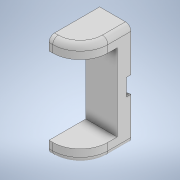
# Autodesk Inventor part: Spine
Saved by Autodesk Inventor 2022 (Build 260153000, 153)
## iProperties
Created: 2022-05-09
Part Number: Spine
Material: Generic
Document SubType Name: Modeling
Designer: dirks
Density: 1 g/cm^3
Appearance: Default
Author: dirks
Autodesk Inventor part; units mm, degrees
ref_plane "YZ Plane" through (0, 0, 0) normal (1, 0, 0) x (0, 1, 0)
ref_plane "XZ Plane" through (0, 0, 0) normal (0, 1, 0) x (-1, 0, 0)
ref_plane "XY Plane" through (0, 0, 0) normal (0, 0, 1) x (1, 0, 0)
sketch "Sketch10" plane through (0, 0, 0) normal (0, 0, 1) x (1, 0, 0)
  line L0 (0, 0) -> (17, 0)
  line L1 (17, 0) -> (17, 55)
  line L2 (17, 55) -> (0, 55)
  line L3 (0, 55) -> (0, 0)
  dimension "d24" = 17
  dimension "d25" = 55
  constraints: 8 end point, 2 parallel, 1 horizontal, 1 perpendicular
  measures "d24" distance of L2.end L1.end
  measures "d25" distance of L1.end L0.end
extrude "Extrusion9" add sketch "Sketch10" along normal blind 5
sketch "Sketch12" plane through (0, 0, 5) normal (0, 0, 1) x (1, 0, 0)
  line L0 (17, 0) -> (17, 55) projected
  line L1 (0, 55) -> (0, 0) projected
  line L2 (0, 0) -> (17, 0) projected
  line L3 (0, 0) -> (17, 0)
  line L4 (17, 0) -> (17, 6)
  line L5 (17, 6) -> (0, 6)
  line L6 (0, 6) -> (0, 0)
  dimension "d32" = 17
  dimension "d33" = 6
  constraints: 8 end point, 2 parallel, 1 horizontal, 1 perpendicular
  measures "d32" distance of L5.end L4.end
  measures "d33" distance of L4.end L3.end
extrude "Extrusion11" add sketch "Sketch12" along normal blind 20
sketch "Sketch13" plane through (0, 0, 0) normal (0, -1, 0) x (1, 0, 0)
  line L0 (0, 0) -> (17, 0) projected
  line L1 (17, 0) -> (17, 25) projected
  line L2 (0, 25) -> (17, 25) projected
  line L3 (0, 0) -> (0, 25) projected
extrude "Extrusion12" add sketch "Sketch13" along normal blind 1
sketch "Sketch14" plane through (0, 0, 5) normal (0, 0, 1) x (1, 0, 0)
  line L0 (17, 6) -> (17, 55) projected
  line L1 (17, 55) -> (0, 55) projected
  line L2 (0, 55) -> (0, 6) projected
  line L3 (17, 55) -> (0, 55) projected
  line L4 (0, 55) -> (17, 55)
  line L5 (17, 55) -> (17, 48)
  line L6 (17, 48) -> (0, 48)
  line L7 (0, 48) -> (0, 55)
  point P0 (0, 0)
  dimension "d38" = 17
  dimension "d39" = 7
  constraints: 8 end point, 2 parallel, 1 horizontal, 1 perpendicular
  measures "d38" distance of L5.end L6.end
  measures "d39" distance of L4.end L5.end
extrude "Extrusion13" add sketch "Sketch14" along normal up to surface (20 mm away)
fillet "Fillet1" radius 15 1 edges at (17, 51.5, 25)
fillet "Fillet2" radius 15 1 edges at (17, 2.5, 25)
fillet "Fillet3" radius 3 3 edges at (1, 55, 25) (17, 55, 5) (12.6066, 55, 20.6066)
fillet "Fillet4" radius 3 3 edges at (12.6066, -1, 20.6066) (1, -1, 25) (17, -1, 5)
sketch "Sketch15" plane through (0, 0, 0) normal (0, 0, -1) x (-1, 0, 0)
  arc A0 (-17, 2) -> (-14, -1) centre (-14, 2) ccw projected
  line L0 (0, -1) -> (-14, -1) projected
  line L1 (0, 55) -> (0, -1) projected
  line L2 (-14, 55) -> (0, 55) projected
  arc A1 (-14, 55) -> (-17, 52) centre (-14, 52) ccw projected
  line L3 (-17, 2) -> (-17, 52) projected
  line L4 (8.7827, 30.0642) -> (-3.3501, 32.1768) projected
  line L5 (-5.4735, 44.3389) -> (-3.3501, 32.1768) projected
  line L6 (-5.4735, 44.3389) -> (-5.8165, 45.0526) projected
  line L7 (-5.8165, 45.0526) -> (-6.5415, 45.6348) projected
  line L8 (-7.5479, 46.0014) -> (-6.5415, 45.6348) projected
  line L9 (-8.6908, 46.1) -> (-7.5479, 46.0014) projected
  line L10 (-8.6908, 46.1) -> (-9.8101, 45.9193) projected
  line L11 (-9.8101, 45.9193) -> (-10.7456, 45.4818) projected
  line L12 (-11.3668, 44.8513) -> (-10.7456, 45.4818) projected
  line L13 (-11.564, 44.3389) -> (-13.6922, 32.1494) projected
  line L14 (-11.3668, 44.8513) -> (-11.564, 44.3389) projected
  line L15 (-13.6922, 32.1494) -> (-25.8859, 30.0262) projected
  line L16 (-25.8859, 23.9358) -> (-13.6462, 21.8046) projected
  line L17 (-3.3041, 21.8692) -> (-5.4356, 9.6611) projected
  line L18 (8.7827, 23.9738) -> (-3.3041, 21.8692) projected
  line L19 (-13.6462, 21.8046) -> (-11.526, 9.6611) projected
  line L20 (-11.526, 9.6611) -> (-11.183, 8.9474) projected
  line L21 (-11.183, 8.9474) -> (-10.458, 8.3652) projected
  line L22 (-10.458, 8.3652) -> (-9.4517, 7.9986) projected
  line L23 (-9.4517, 7.9986) -> (-8.3088, 7.9) projected
  line L24 (-8.3088, 7.9) -> (-7.1895, 8.0807) projected
  line L25 (-7.1895, 8.0807) -> (-6.254, 8.5182) projected
  line L26 (-6.254, 8.5182) -> (-5.6327, 9.1487) projected
  line L27 (-5.4356, 9.6611) -> (-5.6327, 9.1487) projected
  line L28 (0, 48) -> (0, 6) projected
  line L29 (0, 31.5935) -> (-3.3501, 32.1768)
  line L30 (-3.3501, 32.1768) -> (-5.4735, 44.3389)
  line L31 (-3.3041, 21.8692) -> (0, 22.4445)
  line L32 (-3.3041, 21.8692) -> (-5.4356, 9.6611)
  line L33 (-11.526, 9.6611) -> (-13.6462, 21.8046)
  line L34 (-13.6462, 21.8046) -> (-17, 22.3886)
  line L35 (-17, 6) -> (-17, 48) projected
  line L36 (-17, 31.5735) -> (-13.6922, 32.1494)
  line L37 (-13.6922, 32.1494) -> (-11.564, 44.3389)
  arc A2 (-5.4735, 44.3389) -> (-11.564, 44.3389) centre (-8.5188, 42.5301) ccw
  arc A3 (-11.526, 9.6611) -> (-5.4356, 9.6611) centre (-8.4808, 11.4699) ccw
  line L38 (0, 31.5935) -> (0, 22.4445)
  line L39 (-17, 22.3886) -> (-17, 31.5735)
  line L40 (0, 55) -> (0, 52) projected
  line L41 (0, 31.5935) -> (0, 55)
  line L42 (0, 55) -> (-14, 55)
  line L43 (0, 22.4445) -> (0, -1)
  line L44 (-2, -1) -> (-14, -1) projected
  line L45 (-14, -1) -> (0, -1)
  line L46 (-17, 2) -> (-17, 6) projected
  line L47 (-17, 2) -> (-17, 22.3886)
  line L48 (-17, 31.5735) -> (-17, 48)
  arc A4 (-14, 55) -> (-17, 52) centre (-14, 52) ccw
  arc A5 (-17, 2) -> (-14, -1) centre (-14, 2) ccw
  line L49 (-17, 48) -> (-17, 52)
  point P0 (0, 0)
  point P1 (0, 22.4445)
  point P2 (0, 31.5935)
  point P3 (-17, 31.5735)
  constraints: 34 end point, 10 collinear, 10 point on circle, 8 point on line, 4 centre point, 2 perpendicular, 2 tangent, 1 concentric, 1 vertical
extrude "Extrusion14" add sketch "Sketch15" along normal blind 2.5 contours L3 L16 L19 L20 L21 L22 L23 L24 L25 L26 L27 L17 L18 L1 L0 A0 | L3 A1 L2 L1 L4 L5 L6 L7 L8 L9 L10 L11 L12 L14 L13 L15
body "Solid2"
